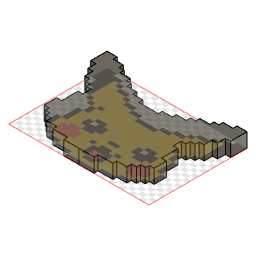
Pik v2 (Autodesk Fusion 360 design; units mm, degrees)
Autodesk Fusion 360 part; units mm, degrees
sketch "pik-sk" plane through (0, 0, 0) normal (0, 0, 1) x (1, 0, 0)
  line L0 (-49.6541, 34.7973) -> (-49.6541, 23.1738)
  line L1 (-49.6541, 23.1738) -> (-45.9923, 23.1738)
  line L2 (-45.9923, 23.1738) -> (-45.9923, 17.5515)
  line L3 (-45.9923, 17.5515) -> (-42.3651, 17.5515)
  line L4 (-42.3651, 17.5515) -> (-42.3651, 11.6579)
  line L5 (-42.3651, 11.6579) -> (-38.829, 11.6579)
  line L6 (-38.829, 11.6579) -> (-38.829, 8.6694)
  line L7 (-38.829, 8.6694) -> (-35.4308, 8.6694)
  line L8 (-35.4308, 8.6694) -> (-35.4308, 5.7405)
  line L9 (-35.4308, 5.7405) -> (-32.068, 5.7405)
  line L10 (-32.068, 5.7405) -> (-32.068, 0.0385)
  line L11 (-32.068, 0.0385) -> (-35.4308, 0.0385)
  line L12 (-35.4308, 0.0385) -> (-35.4308, -11.6953)
  line L13 (-35.4308, -11.6953) -> (-38.9575, -11.6953)
  line L14 (-38.9575, -11.6953) -> (-38.9575, -20.569)
  line L15 (-38.9575, -20.569) -> (-35.4308, -20.569)
  line L16 (-35.4308, -20.569) -> (-35.4308, -23.2957)
  line L17 (-35.4308, -23.2957) -> (-32.0468, -23.2957)
  line L18 (-32.0468, -23.2957) -> (-32.0468, -26.1695)
  line L19 (-32.0468, -26.1695) -> (-28.3803, -26.1695)
  line L20 (-28.3803, -26.1695) -> (-28.3803, -29.3405)
  line L21 (-28.3803, -29.3405) -> (-21.2455, -29.3405)
  line L22 (-21.2455, -29.3405) -> (-21.2455, -32.1152)
  line L23 (-21.2455, -32.1152) -> (-10.7414, -32.1152)
  line L24 (-10.7414, -32.1152) -> (-10.7414, -34.8898)
  line L25 (-10.7414, -34.8898) -> (0.0599, -34.8898)
  line L26 (0, 14.6559) -> (-6.8686, 14.6476)
  line L27 (-6.8686, 14.6476) -> (-6.8721, 17.5432)
  line L28 (-6.8721, 17.5432) -> (-13.9652, 17.5346)
  line L29 (-13.9652, 17.5346) -> (-13.9687, 20.3821)
  line L30 (-13.9687, 20.3821) -> (-21.0302, 20.3735)
  line L31 (-21.0302, 20.3735) -> (-21.0339, 23.4685)
  line L32 (-21.0339, 23.4685) -> (-24.6974, 23.4641)
  line L33 (-24.6974, 23.4641) -> (-24.7009, 26.3367)
  line L34 (-24.7009, 26.3367) -> (-31.8504, 26.3281)
  line L35 (-31.8504, 26.3281) -> (-31.8539, 29.2052)
  line L36 (-31.8539, 29.2052) -> (-35.372, 29.2009)
  line L37 (-35.372, 29.2009) -> (-35.3755, 32.1099)
  line L38 (-35.3755, 32.1099) -> (-42.492, 32.1013)
  line L39 (-42.492, 32.1013) -> (-42.4954, 34.8818)
  line L40 (-42.4954, 34.8818) -> (-49.6541, 34.8818)
  line L41 (-49.6541, 34.8818) -> (-49.6541, 34.7973)
  line L42 (32.0895, 5.8181) -> (32.1032, 0.1161)
  line L43 (35.4451, 8.7551) -> (35.4522, 5.8262)
  line L44 (42.358, 17.6539) -> (42.3722, 11.7604)
  line L45 (31.8186, 29.2822) -> (35.3367, 29.2864)
  line L46 (42.4463, 34.9845) -> (49.605, 35.0018)
  line L47 (21.0163, 20.4244) -> (21.0125, 23.5194)
  line L48 (31.8221, 26.4051) -> (31.8186, 29.2822)
  line L49 (24.6761, 23.5238) -> (24.6726, 26.3964)
  line L50 (42.4497, 32.2039) -> (42.4463, 34.9845)
  line L51 (6.8651, 17.5598) -> (13.9582, 17.5684)
  line L52 (13.9548, 20.4158) -> (21.0163, 20.4244)
  line L53 (0, 14.6559) -> (6.8686, 14.6642)
  line L54 (32.1454, -26.0919) -> (28.4789, -26.1007)
  line L55 (21.3518, -29.289) -> (21.3585, -32.0637)
  line L56 (35.5224, -23.21) -> (32.1385, -23.2181)
  line L57 (35.4944, -11.6095) -> (39.0211, -11.601)
  line L58 (6.8686, 14.6642) -> (6.8651, 17.5598)
  line L59 (35.4522, 5.8262) -> (32.0895, 5.8181)
  line L60 (21.0125, 23.5194) -> (24.6761, 23.5238)
  line L61 (35.3332, 32.1953) -> (42.4497, 32.2039)
  line L62 (42.3722, 11.7604) -> (38.8361, 11.7518)
  line L63 (45.9852, 17.6627) -> (42.358, 17.6539)
  line L64 (49.6052, 34.9173) -> (49.6334, 23.2938)
  line L65 (24.6726, 26.3964) -> (31.8221, 26.4051)
  line L66 (32.1032, 0.1161) -> (35.466, 0.1242)
  line L67 (28.4866, -29.2718) -> (21.3518, -29.289)
  line L68 (35.466, 0.1242) -> (35.4944, -11.6095)
  line L69 (38.8361, 11.7518) -> (38.8433, 8.7633)
  line L70 (38.8433, 8.7633) -> (35.4451, 8.7551)
  line L71 (10.8545, -32.0891) -> (10.8612, -34.8637)
  line L72 (49.605, 35.0018) -> (49.6052, 34.9173)
  line L73 (10.8612, -34.8637) -> (0.0599, -34.8898)
  line L74 (49.6334, 23.2938) -> (45.9716, 23.2849)
  line L75 (32.1385, -23.2181) -> (32.1454, -26.0919)
  line L76 (39.0211, -11.601) -> (39.0425, -20.4747)
  line L77 (35.5158, -20.4832) -> (35.5224, -23.21)
  line L78 (39.0425, -20.4747) -> (35.5158, -20.4832)
  line L79 (35.3367, 29.2864) -> (35.3332, 32.1953)
  line L80 (45.9716, 23.2849) -> (45.9852, 17.6627)
  line L81 (13.9582, 17.5684) -> (13.9548, 20.4158)
  line L82 (28.4789, -26.1007) -> (28.4866, -29.2718)
  line L83 (21.3585, -32.0637) -> (10.8545, -32.0891)
  constraint vertical L0
  constraint perpendicular L0 L1
  constraint perpendicular L1 L2
  constraint perpendicular L2 L3
  constraint perpendicular L3 L4
  constraint perpendicular L4 L5
  constraint perpendicular L5 L6
  constraint perpendicular L6 L7
  constraint perpendicular L7 L8
  constraint perpendicular L8 L9
  constraint perpendicular L9 L10
  constraint perpendicular L10 L11
  constraint perpendicular L9 L12
  constraint perpendicular L12 L13
  constraint perpendicular L9 L14
  constraint perpendicular L14 L15
  constraint perpendicular L15 L16
  constraint perpendicular L16 L17
  constraint perpendicular L17 L18
  constraint perpendicular L18 L19
  constraint perpendicular L17 L20
  constraint perpendicular L20 L21
  constraint perpendicular L17 L22
  constraint perpendicular L22 L23
  constraint perpendicular L23 L24
  constraint perpendicular L24 L25
  constraint perpendicular L26 L27
  constraint perpendicular L28 L29
  constraint perpendicular L29 L30
  constraint perpendicular L30 L31
  constraint perpendicular L29 L32
  constraint perpendicular L32 L33
  constraint perpendicular L33 L34
  constraint perpendicular L34 L35
  constraint perpendicular L35 L36
  constraint perpendicular L34 L37
  constraint perpendicular L37 L38
  constraint perpendicular L38 L39
  constraint perpendicular L0 L40
  constraint perpendicular L40 L41
extrude "Extrude1" add sketch "pik-sk" along normal blind 10
named bodies: "Pik-head"
